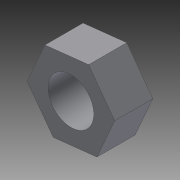
# Autodesk Inventor part: Moer
Saved by Autodesk Inventor 2015 (Build 190159000, 159)
## iProperties
Created: 2016-01-19
Part Number: Moer
Material: Generic
Document SubType Name: Modeling
Designer: david
Density: 1 g/cm^3
Appearance: Default
Mass: 0.291641 g
Surface Area: 3.84109 cm^2
Volume: 0.291641 cm^3
Author: david
Autodesk Inventor part; units mm, degrees
ref_plane "YZ Plane" through (0, 0, 0) normal (1, 0, 0) x (0, 1, 0)
ref_plane "XZ Plane" through (0, 0, 0) normal (0, 1, 0) x (-1, 0, 0)
ref_plane "XY Plane" through (0, 0, 0) normal (0, 0, 1) x (1, 0, 0)
sketch "Sketch1" plane through (0, 0, 0) normal (0, 1, 0) x (-1, 0, 0)
  line L0 (2.3235, -5.2853) -> (-3.4155, -4.6549)
  line L1 (-3.4155, -4.6549) -> (-5.739, 0.6305)
  line L2 (-5.739, 0.6305) -> (-2.3235, 5.2853)
  line L3 (-2.3235, 5.2853) -> (3.4155, 4.6549)
  line L4 (3.4155, 4.6549) -> (5.739, -0.6305)
  line L5 (5.739, -0.6305) -> (2.3235, -5.2853)
  circle A0 centre (0, 0) radius 3
  dimension "d0" = 10
  dimension "d1" = 6
  constraints: 12 end point, 2 coincident, 1 centre point, 13 other
  measures "d0" distance between parallel lines of L0 L3
  measures "d1" diameter of A0
extrude "Extrusion1" add sketch "Sketch1" along normal blind 5
thread "Thread1" size "M6x1" class "6H" standard "ANSI Metric M Profile" full length
body "Solid1"
